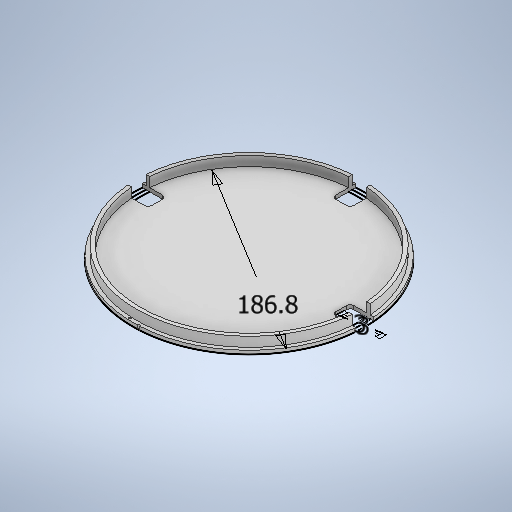
# Autodesk Inventor part: 187mm-CoilForm
Saved by Autodesk Inventor 2025.3 (Build 293356000, 356)
## iProperties
Created: 2025-05-18
Part Number: 187mm-CoilForm
Material: Generic
Document SubType Name: Modeling
Designer: user
Density: 1 g/cm^3
Appearance: Default
Author: user
## iProperties of the stored document 122mm-CoilForm_3DPrint.ipt
Created: 2025-05-18
Part Number: 122mm-CoilForm_3DPrint
Material: Generic
Document SubType Name: Modeling
Designer: user
Density: 1 g/cm^3
Appearance: Default
Author: user
Autodesk Inventor part; units mm, degrees
ref_plane "YZ Plane" through (0, 0, 0) normal (1, 0, 0) x (0, 1, 0)
ref_plane "XZ Plane" through (0, 0, 0) normal (0, 1, 0) x (-1, 0, 0)
ref_plane "XY Plane" through (0, 0, 0) normal (0, 0, 1) x (1, 0, 0)
sketch "Sketch1" plane through (0, 0, 0) normal (0, 1, 0) x (-1, 0, 0)
  circle A0 centre (0, 0) radius 93.4
  circle A1 centre (0, 0) radius 90.4
  circle A2 centre (0, 0) radius 96.4
  dimension "d0" = 186.8
  dimension "d1" = 3
  dimension "d2" = 3
  constraints: 3 centre point, 1 coincident
  measures "d0" diameter of A0
  measures "d1" radial gap between concentric circles of A0 A1
  measures "d2" radial gap between concentric circles of A0 A2
extrude "Extrusion1" add sketch "Sketch1" along normal blind 11 contours A0
extrude "Extrusion2" add sketch "Sketch1" along normal blind 3 contours A2
sketch "Sketch2" plane through (0, 3, 0) normal (0, 1, 0) x (1, 0, 0)
  circle A0 centre (-4.5, -94.2927) radius 1
  circle A1 centre (0, 0) radius 93.4 projected
  circle A2 centre (0, 0) radius 95.4 construction
  circle A3 centre (4.5, -96.2949) radius 1
  dimension "d7" = 2
  dimension "d8" = 4.5
  dimension "d9" = 4.5
  constraints: 3 centre point, 3 tangent, 1 coincident, 1 equal radius
  measures "d7" diameter of A0
  measures "d8" horizontal distance of A0.centre point (0, 0)
  measures "d9" horizontal distance of A3.centre point (0, 0)
extrude "Extrusion3" cut sketch "Sketch2" against normal up to surface (3 mm away) contours A0 | A3
extrude "Extrusion4" add sketch "Sketch1" along normal blind 3 contours A1
sketch "Sketch3" plane through (0, 0, 0) normal (0, -1, 0) x (1, 0, 0)
  line L0 (96.4, -7.5) -> (76.4, -7.5)
  line L1 (76.4, -7.5) -> (76.4, 7.5)
  line L2 (76.4, 7.5) -> (96.4, 7.5)
  line L3 (96.4, 7.5) -> (96.4, -7.5)
  arc A0 (3.5009, 96.3364) -> (5.4987, 96.2431) centre (0, 0) ccw projected
  point P0 (96.4, 0)
  dimension "d14" = 15
  dimension "d15" = 20
  constraints: 8 end point, 2 parallel, 1 horizontal, 1 horizontal alignment, 1 midpoint, 1 perpendicular, 1 tangent
  measures "d14" distance of L2.end L0.start
  measures "d15" distance of L0.start L0.end
extrude "Extrusion5" cut sketch "Sketch3" against normal up to surface (11 mm away) contours L0 A0 L3 | L0 L1 L2 A0 L3 | A0 L2 L3
pattern_circular "Circular Pattern1" count 3 over 180 about axis through (0, -10, 0) along (0, 1, 0) of "Extrusion5"
fillet "Fillet1" radius 3 6 edges at (76.4, 1.5, 7.5) (76.4, 1.5, -7.5) (-76.4, 1.5, 7.5) (-76.4, 1.5, -7.5) (7.5, 1.5, -76.4) (-7.5, 1.5, -76.4)
body "Solid1"
